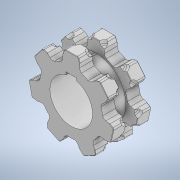
# Autodesk Inventor part: sprocket
Saved by Autodesk Inventor 2021.3 (Build 253353010, 353A)
## iProperties
Created: 2021-05-25
Part Number: sprocket
Material: Generic
Document SubType Name: Modeling
Designer: Lorca
Density: 1 g/cm^3
Appearance: Default
Author: Lorca
Autodesk Inventor part; units mm, degrees
ref_plane "YZ Plane" through (0, 0, 0) normal (1, 0, 0) x (0, 1, 0)
ref_plane "XZ Plane" through (0, 0, 0) normal (0, 1, 0) x (-1, 0, 0)
ref_plane "XY Plane" through (0, 0, 0) normal (0, 0, 1) x (1, 0, 0)
sketch "Sketch1" plane through (0, 0, 0) normal (0, 0, 1) x (1, 0, 0)
  circle A0 centre (0, 0) radius 500
  circle A1 centre (0, 0) radius 350
  line L0 (-120, 350) -> (120, 350)
  line L1 (120, 350) -> (120, 500)
  line L2 (120, 500) -> (-120, 500)
  line L3 (-120, 500) -> (-120, 350)
  circle A2 centre (0, 0) radius 370
  circle A3 centre (0, 0) radius 250
  line L4 (-60, 242.6932) -> (60, 242.6932)
  line L5 (60, 242.6932) -> (60, 272.6932)
  line L6 (60, 272.6932) -> (-60, 272.6932)
  line L7 (-60, 272.6932) -> (-60, 242.6932)
  dimension "d3" = 500
  dimension "d0" = 1000
  dimension "d1" = 700
  dimension "d2" = 240
  dimension "d4" = 120
  dimension "d5" = 30
  constraints: 16 end point, 4 coincident, 4 parallel, 2 centre point, 2 horizontal, 2 perpendicular, 6 other
  measures "d0" diameter of A0
  measures "d1" diameter of A1
  measures "d2" distance of L2.end L1.end
  measures "d4" distance of L6.end L5.end
  measures "d5" distance of L5.end L4.end
extrude "Extrusion1" add sketch "Sketch1" along normal blind 150 contours A1 | A2 L0 | L0 A2
sketch "Sketch2" plane through (0, 0, 0) normal (0, 0, 1) x (1, 0, 0)
  circle A0 centre (0, 0) radius 500
  circle A1 centre (0, 0) radius 350
  line L0 (-100.0095, 349.6696) -> (99.9905, 349.6696)
  line L1 (99.9905, 349.6696) -> (99.9905, 492.4997)
  line L2 (99.9905, 492.4997) -> (-66.9075, 492.4997)
  line L3 (-100.0095, 492.4997) -> (-100.0095, 394.8203)
  circle A2 centre (0, 0) radius 363.6853
  circle A3 centre (0, 0) radius 250
  line L4 (-60, 242.6932) -> (60, 242.6932)
  line L5 (60, 242.6932) -> (60, 272.6932)
  line L6 (60, 272.6932) -> (-60, 272.6932)
  line L7 (-60, 272.6932) -> (-60, 242.6932)
  line L8 (-143.3944, 337.1667) -> (-166.0935, 330.6251)
  circle A4 centre (0, 0) radius 370 projected
  line L9 (-100.0095, 349.6696) -> (-166.0935, 330.6251)
  arc A5 (-143.3944, 337.1667) -> (-100.0095, 394.8203) centre (-160.0095, 394.8203) ccw
  line L10 (-0.0095, 594.1519) -> (-0.0095, 319.1519)
  line L11 (-100.0095, 440.029) -> (-85.7014, 479.3401)
  line L12 (-100.0095, 440.029) -> (-58.1755, 440.029) construction
  arc A6 (-66.9075, 492.4997) -> (-85.7014, 479.3401) centre (-66.9075, 472.4997) ccw
  arc A7 (99.9905, 394.8203) -> (143.3755, 337.1667) centre (159.9905, 394.8203) ccw
  line L13 (99.9905, 440.029) -> (85.6825, 479.3401)
  arc A8 (85.6825, 479.3401) -> (66.8886, 492.4997) centre (66.8886, 472.4997) ccw
  line L14 (0, 0) -> (50, 0)
  point P0 (-119.9276, 357.0484)
  point P1 (119.9008, 357.0574)
  point P2 (-99.9905, 349.6696)
  point P3 (-120.1961, 349.9327)
  point P4 (120.1652, 349.9433)
  dimension "d11" = 500
  dimension "d8" = 1000
  dimension "d9" = 700
  dimension "d10" = 200
  dimension "d12" = 120
  dimension "d13" = 30
  dimension "d17" = 60
  dimension "d19" = 275
  dimension "d20" = 70
  dimension "d21" = 20
  dimension "d22" = 100
  dimension "d23" = 50
  constraints: 30 end point, 8 point on circle, 7 symmetric about line, 6 centre point, 4 coincident, 4 horizontal, 4 parallel, 4 point on line, 4 tangent, 2 perpendicular, 1 equal length, 1 vertical, 10 other
  measures "d8" diameter of A0
  measures "d9" diameter of A1
  measures "d10" distance of L3.start L1.end
  measures "d12" distance of L6.end L5.end
  measures "d13" distance of L5.end L4.end
  measures "d17" radius of A5
  measures "d19" distance of L10.start L10.end
  measures "d20" angle of L12 L11
  measures "d21" radius of A6
  measures "d22" distance between parallel lines of L10 L3
  measures "d23" distance of L14.start L14.end
extrude "Extrusion2" add sketch "Sketch2" along normal blind 150 contours L1 A4 L10 L2 A8 L13 | L11 A6 L2 L10 A4 A5 L3 | A7 A4 L1
pattern_circular "Circular Pattern1" count 7 over 360 about axis through (0, 0, -10) along (0, 0, 1) of "Extrusion2"
sketch "Sketch3" plane through (0, 0, 150) normal (0, 0, 1) x (1, 0, 0)
  line L0 (-100.0095, 440.029) -> (-100.0095, 394.8203) projected
  line L1 (66.8886, 492.4997) -> (-66.9075, 492.4997) projected
  line L2 (-100.0095, 440.029) -> (-40.0095, 440.029)
  line L3 (-40.0095, 440.029) -> (-40.0095, 492.4997)
  line L4 (-40.0095, 492.4997) -> (-100.0095, 492.4997)
  line L5 (-100.0095, 492.4997) -> (-100.0095, 440.029)
  line L6 (-100.0095, 492.4997) -> (-55.0095, 492.4997)
  line L7 (-55.0095, 492.4997) -> (-55.0095, 452.4997)
  line L8 (-55.0095, 452.4997) -> (-100.0095, 452.4997)
  line L9 (-100.0095, 452.4997) -> (-100.0095, 492.4997)
  line L10 (-100.0095, 440.029) -> (-64.8202, 449.7808)
  line L11 (-51.4348, 462.032) -> (-40.0095, 492.4997)
  arc A0 (-64.8202, 449.7808) -> (-51.4348, 462.032) centre (-70.1614, 469.0544) ccw
  point P0 (0, 0)
  dimension "d27" = 60
  dimension "d28" = 45
  dimension "d29" = 40
  dimension "d30" = 20
  constraints: 20 end point, 4 parallel, 3 point on line, 2 horizontal, 2 perpendicular, 2 point on circle, 2 tangent, 1 centre point
  measures "d27" distance of L4.end L3.end
  measures "d28" distance of L7.end L8.end
  measures "d29" distance of L6.end L7.end
  measures "d30" radius of A0
revolve "Revolution1" cut sketch "Sketch3" angle 360 about axis through (-100.0095, 440.029, 150) along (0, -1, 0) contours L11 A0 L7 L1 | L7 A0 L8 L5 L4 L1 | L5 L8 A0 L10
mirror "Mirror1" about plane through (0, 0, 0) normal (1, 0, 0) of "Revolution1"
pattern_circular "Circular Pattern2" count 7 over 360 about axis through (0, 0, -10) along (0, 0, 1) of "Revolution1", "Mirror1"
sketch "Sketch4" plane through (0, 0, 0) normal (0, 0, 1) x (1, 0, 0)
  circle A0 centre (0, 0) radius 500
  circle A1 centre (0, 0) radius 350
  line L0 (-100.0095, 349.6696) -> (99.9905, 349.6696)
  line L1 (99.9905, 349.6696) -> (99.9905, 492.4997)
  line L2 (99.9905, 492.4997) -> (-66.9075, 492.4997)
  line L3 (-100.0095, 492.4997) -> (-100.0095, 394.8203)
  circle A2 centre (0, 0) radius 363.6853
  circle A3 centre (0, 0) radius 250
  line L4 (-60, 242.6932) -> (60, 242.6932)
  line L5 (60, 242.6932) -> (60, 272.6932)
  line L6 (60, 272.6932) -> (-60, 272.6932)
  line L7 (-60, 272.6932) -> (-60, 242.6932)
  line L8 (-143.3944, 337.1667) -> (-166.0935, 330.6251)
  line L9 (-100.0095, 349.6696) -> (-166.0935, 330.6251)
  arc A4 (-143.3944, 337.1667) -> (-100.0095, 394.8203) centre (-160.0095, 394.8203) ccw
  line L10 (-0.0095, 594.1519) -> (-0.0095, 319.1519)
  line L11 (-100.0095, 440.029) -> (-85.7014, 479.3401)
  line L12 (-100.0095, 440.029) -> (-58.1755, 440.029) construction
  arc A5 (-66.9075, 492.4997) -> (-85.7014, 479.3401) centre (-66.9075, 472.4997) ccw
  arc A6 (99.9905, 394.8203) -> (143.3755, 337.1667) centre (159.9905, 394.8203) ccw
  line L13 (99.9905, 440.029) -> (85.6825, 479.3401)
  arc A7 (85.6825, 479.3401) -> (66.8886, 492.4997) centre (66.8886, 472.4997) ccw
  line L14 (0, 0) -> (50, 0)
  point P0 (-119.9276, 357.0484)
  point P1 (119.9008, 357.0574)
  point P2 (-99.9905, 349.6696)
  point P3 (-120.1961, 349.9327)
  point P4 (120.1652, 349.9433)
  point P5 (-15.2032, 349.6696)
  point P6 (15.2032, 349.6696)
  dimension "d38" = 500
  dimension "d35" = 1000
  dimension "d36" = 700
  dimension "d37" = 200
  dimension "d39" = 120
  dimension "d40" = 30
  dimension "d41" = 60
  dimension "d42" = 275
  dimension "d43" = 70
  dimension "d44" = 20
  dimension "d45" = 100
  dimension "d46" = 50
  constraints: 30 end point, 8 point on circle, 7 symmetric about line, 6 centre point, 4 coincident, 4 horizontal, 4 parallel, 4 point on line, 4 tangent, 2 perpendicular, 1 equal length, 1 vertical, 11 other
  measures "d35" diameter of A0
  measures "d36" diameter of A1
  measures "d37" distance of L3.start L1.end
  measures "d39" distance of L6.end L5.end
  measures "d40" distance of L5.end L4.end
  measures "d41" radius of A4
  measures "d42" distance of L10.start L10.end
  measures "d43" angle of L12 L11
  measures "d44" radius of A5
  measures "d45" distance between parallel lines of L10 L3
  measures "d46" distance of L14.start L14.end
extrude "Extrusion3" add sketch "Sketch4" along normal blind 220 contours A1 L0
mirror "Mirror2" about plane through (0, -0.1652, 220) normal (0, 0, 1)
chamfer "Chamfer1" distance 5 angle 45 84 edges at (0, 492.4997, 150) (-0.0095, 492.4997, 0) (-78.3791, 488.8827, 0) (-92.8554, 459.6845, 0) (78.3602, 488.8827, 0) (92.8365, 459.6845, 0) (0, 492.4997, 290) (-0.0095, 492.4997, 440) (-78.3791, 488.8827, 440) (-92.8554, 459.6845, 440) (78.3602, 488.8827, 440) (92.8365, 459.6845, 440) (-385.0576, 307.0611, 0) (-431.0924, 243.5341, 0) (-417.2902, 214.0113, 0) (-333.3671, 366.0778, 0) (-301.5132, 359.1911, 0) (-385.0517, 307.0685, 150) (-385.0517, 307.0685, 290) (-385.0576, 307.0611, 440) (-431.0924, 243.5341, 440) (-417.2902, 214.0113, 440) (-333.3671, 366.0778, 440) (-301.5132, 359.1911, 440) (385.0458, 307.0759, 440) (333.3553, 366.0926, 440) (301.5014, 359.2059, 440) (431.0806, 243.5489, 440) (417.2785, 214.0261, 440) (480.1538, -109.5823, 440) (494.0664, -32.3727, 440) (468.8216, -11.7621, 440) (459.1886, -185.1821, 440) (427.5012, -192.7983, 440) (213.6961, -443.7228, 440) (282.7354, -406.4607, 440) (283.1095, -373.873, 440) (141.5182, -474.4673, 440) (115.8068, -454.4417, 440) (-213.6791, -443.731, 440) (-141.5011, -474.4755, 440) (-115.7898, -454.4499, 440) (-282.7183, -406.4689, 440) (-283.0925, -373.8812, 440) (-480.1496, -109.6007, 440) (-459.1844, -185.2006, 440) (-427.497, -192.8168, 440) (-494.0622, -32.3911, 440) (-468.8173, -11.7805, 440) (-480.1496, -109.6007, 0) (-459.1844, -185.2006, 0) (-427.497, -192.8168, 0) (-494.0622, -32.3911, 0) (-468.8173, -11.7805, 0) (-213.6791, -443.731, 0) (-141.5011, -474.4755, 0) (-115.7898, -454.4499, 0) (-282.7183, -406.4689, 0) (-283.0925, -373.8812, 0) (213.6961, -443.7228, 0) (282.7354, -406.4607, 0) (283.1095, -373.873, 0) (141.5182, -474.4673, 0) (115.8068, -454.4417, 0) (480.1538, -109.5823, 0) (494.0664, -32.3727, 0) (468.8216, -11.7621, 0) (459.1886, -185.1821, 0) (427.5012, -192.7983, 0) (385.0458, 307.0759, 0) (333.3553, 366.0926, 0) (301.5014, 359.2059, 0) (431.0806, 243.5489, 0) (417.2785, 214.0261, 0) (480.1517, -109.5915, 290) (480.1517, -109.5915, 150) (213.6876, -443.7269, 290) (213.6876, -443.7269, 150) (-213.6876, -443.7269, 290) (-213.6876, -443.7269, 150) (-480.1517, -109.5915, 150) (-480.1517, -109.5915, 290) (385.0517, 307.0685, 150) (385.0517, 307.0685, 290)
body "Solid1"
